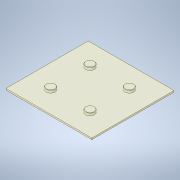
# Autodesk Inventor part: Bottom Surface
Saved by Autodesk Inventor 2022 (Build 260153000, 153)
## iProperties
Created: 2021-03-04
Part Number: Bottom Surface
Material: Polytetrafluoroethylene
Document SubType Name: Modeling
Designer: caleb
Density: 2.02 g/cm^3
Appearance: Smooth - Ivory
Author: caleb
Autodesk Inventor part; units mm, degrees
ref_plane "YZ Plane" through (0, 0, 0) normal (1, 0, 0) x (0, 1, 0)
ref_plane "XZ Plane" through (0, 0, 0) normal (0, 1, 0) x (-1, 0, 0)
ref_plane "XY Plane" through (0, 0, 0) normal (0, 0, 1) x (1, 0, 0)
sketch "Sketch1" plane through (0, 0, 0) normal (0, 1, 0) x (-1, 0, 0)
  line L0 (-24, 23) -> (24, 23)
  line L1 (24, 23) -> (24, -23)
  line L2 (24, -23) -> (-24, -23)
  line L3 (-24, -23) -> (-24, 23)
  line L4 (-24, 23) -> (24, -23) construction
  line L5 (24, 23) -> (-24, -23) construction
  point P0 (0, 0)
  dimension "d0" = 46
  dimension "d1" = 48
  constraints: 12 end point, 2 midpoint, 2 parallel, 1 horizontal, 1 perpendicular
  measures "d0" distance of L0.end L1.end
  measures "d1" distance of L0.start L0.end
extrude "Extrusion1" add sketch "Sketch1" along normal blind 2
sketch "Sketch2" plane through (0, 2, 0) normal (0, 1, 0) x (1, 0, 0)
  circle A0 centre (-11, -11) radius 2.5
  line L0 (-24, 23) -> (-24, -23) projected
  line L1 (-24, -23) -> (24, -23) projected
  circle A1 centre (-11, 11) radius 2.5
  circle A2 centre (11, -11) radius 2.5
  circle A3 centre (11, 11) radius 2.5
  point P0 (0, 0)
  dimension "d4" = 5
  dimension "d17" = 11
  dimension "d18" = 11
  dimension "d21" = 22
  dimension "d24" = 22
  constraints: 4 centre point, 1 horizontal, 1 vertical, 6 other
  measures "d4" diameter of A0
  measures "d17" horizontal distance of point (0, 0) A0.centre
  measures "d18" horizontal distance of A0.centre point (0, 0)
  measures "d21" distance of A0.centre A1.centre
  measures "d24" distance of A0.centre A2.centre
extrude "Extrusion2" add sketch "Sketch2" along normal blind 1.5
fillet "Fillet1" radius 0.2 1 edges at (-13.5, 3.5, 11)
fillet "Fillet2" radius 0.2 3 edges at (-13.5, 3.5, -11) (8.5, 3.5, -11) (8.5, 3.5, 11)
sketch "Sketch3" plane through (0, 0, 0) normal (0, -1, 0) x (1, 0, 0)
  line L0 (24, -23) -> (-24, -23) projected
  line L1 (-24, 23) -> (24, 23)
  line L2 (24, 23) -> (24, -23)
  line L3 (24, -23) -> (-24, -23)
  line L4 (-24, -23) -> (-24, 23)
  line L5 (-24, 23) -> (24, -23) construction
  line L6 (24, 23) -> (-24, -23) construction
  line L7 (-21.925, 21.3) -> (21.925, 21.3)
  line L8 (21.925, 21.3) -> (21.925, -21.3)
  line L9 (21.925, -21.3) -> (-21.925, -21.3)
  line L10 (-21.925, -21.3) -> (-21.925, 21.3)
  line L11 (-21.925, 21.3) -> (21.925, -21.3) construction
  line L12 (21.925, 21.3) -> (-21.925, -21.3) construction
  point P0 (0, 0)
  dimension "d12" = 43.85
  dimension "d13" = 42.6
  constraints: 24 end point, 4 midpoint, 4 parallel, 2 horizontal, 2 perpendicular
  measures "d12" distance of L7.start L7.end
  measures "d13" distance of L7.end L8.end
extrude "Extrusion3" cut sketch "Sketch3" against normal blind 1
fillet "Fillet3" radius 0.2 16 edges at (24, 1, 0) (21.925, 0, 0) (21.925, 0.5, 21.3) (0, 0, 21.3) (0, 1, 23) (-21.925, 0, 0) (-24, 1, 0) (-21.925, 0.5, -21.3) (0, 0, -21.3) (21.925, 0.5, -21.3) (0, 1, -23) (-21.925, 0.5, 21.3) (-24, 1.5, 23) (-24, 1.5, -23) (24, 1.5, -23) (24, 1.5, 23)
body "Solid1"
